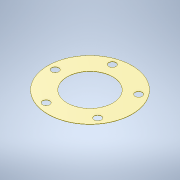
# Autodesk Inventor part: Part7
Saved by Autodesk Inventor 2020 (Build 240168000, 168)
## iProperties
Created: 2021-10-14
Part Number: Part7
Material: Nylon 6/6
Document SubType Name: Modeling
Designer: simon.erikssonwestl
Density: 1.13 g/cm^3
Appearance: Nylon 6
Author: simon.erikssonwestl
Autodesk Inventor part; units mm, degrees
ref_plane "YZ Plane" through (0, 0, 0) normal (1, 0, 0) x (0, 1, 0)
ref_plane "XZ Plane" through (0, 0, 0) normal (0, 1, 0) x (-1, 0, 0)
ref_plane "XY Plane" through (0, 0, 0) normal (0, 0, 1) x (1, 0, 0)
sketch "Sketch1" plane through (0, 0, 0) normal (0, 1, 0) x (-1, 0, 0)
  circle A0 centre (0, 0) radius 17.5
  circle A1 centre (0, 0) radius 9.5
  dimension "d0" = 35
  dimension "d1" = 19
  constraints: 2 centre point, 2 coincident
  measures "d0" diameter of A0
  measures "d1" diameter of A1
extrude "Extrusion1" add sketch "Sketch1" along normal mid plane 0.1
sketch "Sketch2" plane through (0, 0.05, 0) normal (0, 1, 0) x (1, 0, 0)
  circle A0 centre (-14.5, 0) radius 1.5
  circle A1 centre (-4.4807, -13.7903) radius 1.5
  circle A2 centre (11.7307, -8.5229) radius 1.5
  circle A3 centre (11.7307, 8.5229) radius 1.5
  circle A4 centre (-4.4807, 13.7903) radius 1.5
  point P0 (0, 0)
  dimension "d4" = 3
  dimension "d5" = 0
  dimension "d6" = 14.5
  dimension "d9" = 360
  constraints: 5 centre point, 11 other
  measures "d4" diameter of A0
  measures "d5" vertical distance of point (0, 0) A0.centre
  measures "d6" distance of point (0, 0) A0.centre
extrude "Extrusion2" cut sketch "Sketch2" against normal through all
body "Solid1"
